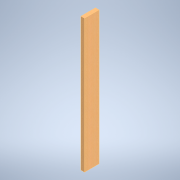
# Autodesk Inventor part: pull Up beams
Saved by Autodesk Inventor 2021 (Build 250183000, 183)
## iProperties
Created: 2020-12-20
Part Number: pull Up beams
Material: Wood (Oak)
Document SubType Name: Modeling
Designer: Jawad
Density: 0.76 g/cm^3
Appearance: Yellow Pine - Solid Stained Dark No Gloss
Author: Jawad
Autodesk Inventor part; units mm, degrees
ref_plane "YZ Plane" through (0, 0, 0) normal (1, 0, 0) x (0, 1, 0)
ref_plane "XZ Plane" through (0, 0, 0) normal (0, 1, 0) x (-1, 0, 0)
ref_plane "XY Plane" through (0, 0, 0) normal (0, 0, 1) x (1, 0, 0)
sketch "Sketch1" plane through (0, 0, 0) normal (0, 1, 0) x (-1, 0, 0)
  line L0 (127.8428, 167.3913) -> (59.0928, 167.3913)
  line L1 (59.0928, 167.3913) -> (59.0928, -107.6087)
  line L2 (59.0928, -107.6087) -> (127.8428, -107.6087)
  line L3 (127.8428, -107.6087) -> (127.8428, 167.3913)
  point P0 (0, 0)
  dimension "d0" = 275
  dimension "d1" = 68.75
  constraints: 8 end point, 2 parallel, 1 horizontal, 1 perpendicular
  measures "d0" distance of L2.end L0.start
  measures "d1" distance of L1.end L2.end
extrude "Extrusion1" add sketch "Sketch1" along normal blind 2500
equation "\"d1\" = 0.25 * d0"
body "Solid1"
